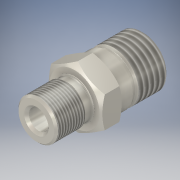
# Autodesk Inventor part: Деталь1
Saved by Autodesk Inventor 2019.3 (Build 233278000, 278)
## iProperties
Created: 2020-04-17
Part Number: Деталь1
Material: Вода
Document SubType Name: Modeling
Designer: Admin
Density: 0.9983 g/cm^3
Appearance: Титан
Author: Admin
Autodesk Inventor part; units mm, degrees
ref_plane "YZ Plane" through (0, 0, 0) normal (1, 0, 0) x (0, 1, 0)
ref_plane "XZ Plane" through (0, 0, 0) normal (0, 1, 0) x (-1, 0, 0)
ref_plane "XY Plane" through (0, 0, 0) normal (0, 0, 1) x (1, 0, 0)
sketch "Эскиз1" plane through (0, 0, 0) normal (0, 0, 1) x (1, 0, 0)
  line L0 (0, 26) -> (22.5167, 13)
  line L1 (22.5167, 13) -> (22.5167, -13)
  line L2 (22.5167, -13) -> (0, -26)
  line L3 (0, -26) -> (-22.5167, -13)
  line L4 (-22.5167, -13) -> (-22.5167, 13)
  line L5 (-22.5167, 13) -> (0, 26)
  point P0 (0, 0)
  point P1 (0, 0)
  dimension "d0" = 52
  constraints: 12 end point, 1 coincident, 1 vertical alignment, 13 other
  measures "d0" distance of L2.end L0.start
extrude "Выдавливание1" add sketch "Эскиз1" along normal blind 18
sketch "Эскиз2" plane through (0, 0, 18) normal (0, 0, 1) x (1, 0, 0)
  circle A0 centre (0, 0) radius 16.6245
  dimension "d3" = 33.249
  constraints: 1 centre point, 1 coincident
  measures "d3" diameter of A0
sketch "Эскиз3" plane through (0, 0, 0) normal (0, 0, -1) x (-1, 0, 0)
  circle A0 centre (0, 0) radius 21
  dimension "d4" = 42
  constraints: 1 centre point, 1 coincident
  measures "d4" diameter of A0
extrude "Выдавливание2" add sketch "Эскиз3" along normal blind 40
extrude "Выдавливание3" add sketch "Эскиз2" along normal blind 32
sketch "Эскиз4" plane through (0, 0, 50) normal (0, 0, 1) x (1, 0, 0)
  circle A0 centre (0, 0) radius 8.25
  dimension "d9" = 16.5
  constraints: 1 centre point, 1 coincident
  measures "d9" diameter of A0
sketch "Эскиз5" plane through (0, 0, -40) normal (0, 0, -1) x (-1, 0, 0)
  point P0 (0, 0)
  point P1 (0, 0)
  constraints: 1 coincident
hole "Отверстие1" at (0, 0, -40) direction (0, 0, 1) diameter 29.211 depth 32 thread size "M33x3.5" class "6H" standard "ISO Metric profile"
extrude "Выдавливание4" cut sketch "Эскиз4" against normal through all
thread "Резьба1" size "G33.249x2.309" designation "G 1" class "A" standard "ISO Pipe Threads" full length
thread "Резьба2" size "M42x4.5" class "6g" standard "ANSI Metric M Profile" length 30
sketch "Эскиз6" plane through (0, 0, 0) normal (1, 0, 0) x (0, 1, 0)
  line L0 (26, 0) -> (26, 18) projected
  line L1 (13, 18) -> (26, 18) projected
  line L2 (26, 0) -> (13, 0) projected
  line L3 (26, 15.1132) -> (21, 18)
  line L4 (26, 2.8868) -> (21, 0)
  line L5 (0, -58) -> (0, 68) projected
  point P0 (0, 0)
  dimension "d25" = 21
  dimension "d26" = 30
  dimension "d27" = 30
  constraints: 4 end point, 4 point on line, 1 vertical alignment
  measures "d25" horizontal distance of point (0, 0) L3.end
  measures "d26" angle of L1 L3
  measures "d27" angle of L2 L4
revolve "Вращение1" cut sketch "Эскиз6" angle 360 about axis through (0, 0, -10) along (0, 0, 1)
sketch "Эскиз7" plane through (0, 0, 0) normal (0, 1, 0) x (-1, 0, 0)
  line L0 (-16.6245, 18) -> (-16.6245, 50) projected
  line L1 (21, 18) -> (-21, 18) projected
  line L2 (-15.6464, 24.7464) -> (-16.6245, 25.7245)
  line L3 (-15.5, 24.3929) -> (-15.5, 19.6)
  line L4 (-16.6245, 18) -> (16.6245, 18) projected
  arc A0 (-17.1, 18) -> (-15.5, 19.6) centre (-17.1, 19.6) ccw
  arc A1 (-15.5, 24.3929) -> (-15.6464, 24.7464) centre (-16, 24.3929) ccw
  line L5 (15.5, -9.6) -> (15.5, -12.5858)
  line L6 (15.2071, -13.2929) -> (14.6055, -13.8945)
  line L7 (14.6055, -8) -> (14.6055, -40) projected
  line L8 (-14.6055, -8) -> (14.6055, -8) projected
  line L9 (13.9, -8) -> (13.4971, -8)
  arc A2 (15.5, -9.6) -> (13.9, -8) centre (13.9, -9.6) ccw
  arc A3 (15.2071, -13.2929) -> (15.5, -12.5858) centre (14.5, -12.5858) ccw
  line L10 (-21, -10) -> (-20.5, -10)
  line L11 (-19.5, -11) -> (-19.5, -13)
  line L12 (-19.6464, -13.3536) -> (-21, -14.7071)
  arc A4 (-19.5, -11) -> (-20.5, -10) centre (-20.5, -11) ccw
  arc A5 (-19.6464, -13.3536) -> (-19.5, -13) centre (-20, -13) ccw
  line L13 (-21, 0) -> (-21, -40) projected
  line L14 (14.6055, -13.8945) -> (13.4971, -8)
  line L15 (-21, -10) -> (-21, -14.7071)
  line L16 (-16.6245, 25.7245) -> (-17.1, 18)
  line L17 (0, -58) -> (0, 68) projected
  point P0 (0, 0)
  point P1 (-15.5, 24.6)
  point P2 (-15.5, 18)
  point P3 (15.5, -8)
  point P4 (15.5, -13)
  dimension "d29" = 31
  dimension "d30" = 45
  dimension "d31" = 1.6
  dimension "d32" = 5
  dimension "d33" = 0.5
  dimension "d34" = 31
  dimension "d35" = 45
  dimension "d36" = 1.6
  dimension "d37" = 5
  dimension "d38" = 1
  dimension "d39" = 45
  dimension "d40" = 1
  dimension "d41" = 0.5
  dimension "d42" = 3
  dimension "d43" = 30
  dimension "d44" = 39
  constraints: 22 end point, 13 point on line, 12 point on circle, 11 tangent, 6 centre point, 2 vertical, 1 collinear, 1 horizontal, 1 perpendicular, 1 vertical alignment
  measures "d29" diameter of point (0, 0) L3
  measures "d30" angle of L0 L2
  measures "d31" radius of A0
  measures "d32" distance of L3.end point (-15.5, 24.6)
  measures "d33" radius of A1
  measures "d34" diameter of point (0, 0) L5
  measures "d35" angle of L7 L6
  measures "d36" radius of A2
  measures "d37" distance from line of L8 point (15.5, -13)
  measures "d38" radius of A3
  measures "d39" angle of L11 L12
  measures "d40" radius of A4
  measures "d41" radius of A5
  measures "d42" distance from line of L10 L11.end
  measures "d43" distance of L13.end L10.start
  measures "d44" diameter of point (0, 0) L11
revolve "Вращение2" cut sketch "Эскиз7" angle 360 about axis through (0, 0, -10) along (0, 0, 1) contours A0 L16 L0 | L0 L2 A1 L3 A0 | L5 A3 L6 L7 A2 | L7 L14 L8 A2 | L10 A4 L11 A5 L12 L13
chamfer "Фаска1" distance 1.6 angle 45 1 edges at (-16.6245, 0, 50)
chamfer "Фаска2" distance 2 angle 45 2 edges at (-8.25, 0, 50) (21, 0, -40)
chamfer "Фаска3" distance 3 angle 45 1 edges at (0, -14.6055, -40)
